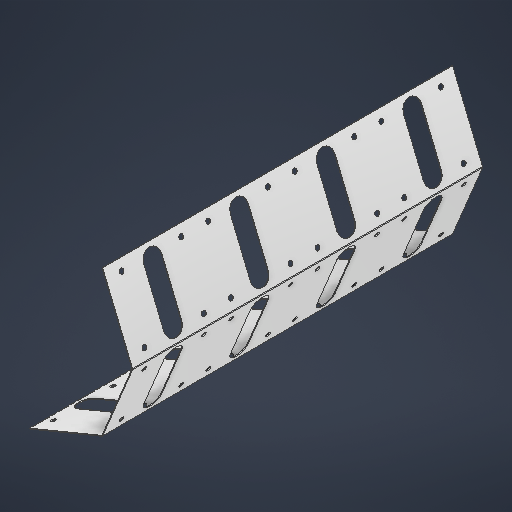
# Autodesk Inventor part: DMF 01 14 Барабан Лист прав брт v2.1
Saved by Autodesk Inventor 2026.2 (Build 302298010, 298A)
## iProperties
Created: 2024-04-28
Part Number: DMF 01 14 Барабан Лист прав брт v2.1
Material: Stainless Steel AISI 304
Document SubType Name: Sheet Metal
Designer: pokla
Density: 8 g/cm^3
Appearance: Chrome - Satin
Sheet Metal Rule: Default
Flat Pattern Width: 65.4696 cm
Flat Pattern Length: 97 cm
Flat Pattern Area: 6350.55 cm^2
Sheet Metal Width: 654,696 mm
Sheet Metal Length: 970,000 mm
Sheet Metal Area: 635055,159 mm^2
Stock Number: Барабан_Лист_Правый_Борт
d174: 145,000 mm
d175: 50,000 mm
Author: pokla
Autodesk Inventor part; units mm, degrees
ref_plane "YZ Plane" through (0, 0, 0) normal (1, 0, 0) x (0, 1, 0)
ref_plane "XZ Plane" through (0, 0, 0) normal (0, 1, 0) x (-1, 0, 0)
ref_plane "XY Plane" through (0, 0, 0) normal (0, 0, 1) x (1, 0, 0)
sketch "Sketch2" plane through (0, 0, 0) normal (0, 0, 1) x (1, 0, 0)
  line L0 (0, 286.833933) -> (202.822219, 202.822219) construction
  line L1 (202.822219, 202.822219) -> (286.833933, 0) construction
  line L2 (286.833933, 0) -> (202.822219, -202.822219) construction
  line L3 (202.822219, -202.822219) -> (0, -286.833933) construction
  line L4 (0, -286.833933) -> (-202.822219, -202.822219) construction
  line L5 (-202.822219, -202.822219) -> (-286.833933, 0) construction
  line L6 (-286.833933, 0) -> (-202.822219, 202.822219) construction
  line L7 (-202.822219, 202.822219) -> (0, 286.833933) construction
  line L8 (203.166634, 201.990728) -> (286.199882, 1.530734)
  line L9 (286.199882, -1.530734) -> (203.45627, -201.291485)
  arc A0 (286.199882, -1.530734) -> (286.199882, 1.530734) centre (282.504364, 0) ccw
  line L10 (201.291485, -203.45627) -> (0.831492, -286.489518)
  arc A1 (201.291485, -203.45627) -> (203.45627, -201.291485) centre (199.760752, -199.760752) ccw
  line L11 (286.833933, 0) -> (286.199882, 1.530734) construction
  line L12 (286.199882, 1.530734) -> (287.730616, 2.164784) construction
  line L13 (287.730616, 2.164784) -> (288.364667, 0.634051) construction
  line L14 (288.364667, 0.634051) -> (286.833933, 0) construction
  line L15 (1.530734, 286.199882) -> (0, 286.833933) construction
  line L16 (0, 286.833933) -> (0.634051, 288.364667) construction
  line L17 (0.634051, 288.364667) -> (2.164784, 287.730616) construction
  line L18 (2.164784, 287.730616) -> (1.530734, 286.199882) construction
  point P0 (0, 0)
  point P1 (0, 0)
  dimension "d56" = 530
  dimension "d58" = 4
  dimension "d69" = 0.9
  dimension "d70" = 4
  dimension "d149" = 0.9
  measures "d56" distance between parallel lines of L6 L2
  measures "d58" radius of A0
  measures "d69" distance of L3.end L10.end
  measures "d70" radius of A1
  measures "d149" distance of L0.end L8.start
contour flange "Contour Flange2" sketch "Sketch2" thickness 2 bend radius 2 width 970 along (0, 0, 1) mid plane no both sides no wall seen from (244.683258, 101.760731, 0) lies toward (-0.9238795, -0.3826834, 0) curves L8 A0 L9 A1 L10
bend "Bend2"
corner "Corner2"
sketch "Sketch13" plane through (203.45627, -201.291485, 970) normal (0.9238795, -0.3826834, 0) x (0, 0, -1)
  line L0 (0, 0) -> (0, 216.21948)
  line L1 (970, 216.21948) -> (970, 0)
  line L2 (820, 180.60974) -> (870, 180.60974) construction
  line L3 (870, 180.60974) -> (870, 35.60974)
  line L4 (870, 35.60974) -> (820, 35.60974) construction
  line L5 (820, 35.60974) -> (820, 180.60974)
  line L6 (820, 180.60974) -> (870, 35.60974) construction
  line L7 (870, 180.60974) -> (820, 35.60974) construction
  arc A0 (870, 180.60974) -> (820, 180.60974) centre (845, 180.60974) ccw
  arc A1 (820, 35.60974) -> (870, 35.60974) centre (845, 35.60974) ccw
  circle A2 centre (762.5, 190.60974) radius 5.5 construction
  circle A3 centre (927.5, 190.60974) radius 5.5 construction
  line L8 (845, 180.60974) -> (845, 35.60974) construction
  line L9 (870, 108.10974) -> (820, 108.10974) construction
  circle A4 centre (762.5, 25.60974) radius 5.5 construction
  circle A5 centre (927.5, 25.60974) radius 5.5 construction
  circle A6 centre (762.5, 190.60974) radius 6.5
  circle A7 centre (845, 190.60974) radius 6.5 construction
  circle A8 centre (845, 25.60974) radius 6.5 construction
  circle A9 centre (762.5, 25.60974) radius 6.5
  circle A10 centre (927.5, 25.60974) radius 6.5
  circle A11 centre (927.5, 190.60974) radius 6.5
  point P0 (970, 108.10974)
  point P1 (0, 108.10974)
  point P2 (845, 108.10974)
  point P3 (845, 108.10974)
  point P4 (970, 108.10974)
  dimension "d166" = 145
  dimension "d167" = 50
  dimension "d168" = 165
  dimension "d169" = 165
  dimension "d170" = 11
  dimension "d171" = 13
  dimension "d172" = 13
  dimension "d173" = 165
  dimension "d176" = 100
  constraints: 16 end point, 12 centre point, 7 midpoint, 4 coincident, 4 point on circle, 4 tangent, 3 equal radius, 2 parallel, 2 point on line, 1 horizontal, 1 horizontal alignment, 1 perpendicular, 1 vertical, 4 other
  measures "d166" distance of L2.end L3.end
  measures "d167" distance of L2.start L2.end
  measures "d168" distance of A3.centre A2.centre
  measures "d169" distance of A5.centre A3.centre
  measures "d170" diameter of A2
  measures "d171" diameter of A6
  measures "d172" diameter of A7
  measures "d173" distance of A8.centre A7.centre
  measures "d176" distance between parallel lines of L1 L3
extrude "Cut2" cut sketch "Sketch13" against normal blind 2
pattern_linear "Rectangular Pattern4" count 4 spacing 240 along (0, 0, 1) of "Cut2"
pattern_circular "Circular Pattern3" count 3 over 90 about axis through (0, 0, -10) along (0, 0, 1) of "Cut2", "Rectangular Pattern4" both ways yes
equation "\"d56\" = Барабан_размер_по_плоскостям"
equation "\"d58\" = BendRadius + Thickness"
equation "\"d69\" = Барабан_отступ_развертки"
equation "\"d70\" = BendRadius + Thickness"
equation "\"d25\" = Thickness"
equation "\"d26\" = BendReliefWidth"
equation "\"d27\" = BendReliefDepth"
equation "\"d28\" = MinimumRemnant"
equation "\"d29\" = TransitionRadius"
equation "\"d31\" = BendRadius"
equation "\"d33\" = CornerReliefSize"
equation "\"d34\" = GapSize"
equation "\"d35\" = JacobiRadiusSize"
equation "\"BendRadius\" = Thickness"
equation "\"BendReliefWidth\" = Thickness"
equation "\"BendReliefDepth\" = 0.5 * Thickness"
equation "\"CornerReliefSize\" = 4 * Thickness"
equation "\"MinimumRemnant\" = 2 * Thickness"
equation "\"TransitionRadius\" = BendRadius"
equation "\"JacobiRadiusSize\" = BendRadius"
equation "\"GapSize\" = Thickness"
equation "\"d174\" = 145"
equation "\"Барабан_размер_по_плоскостям\" = 530"
equation "\"Thickness\" = 2"
equation "\"Барабан_отступ_развертки\" = 0.9"
body "Solid2"
